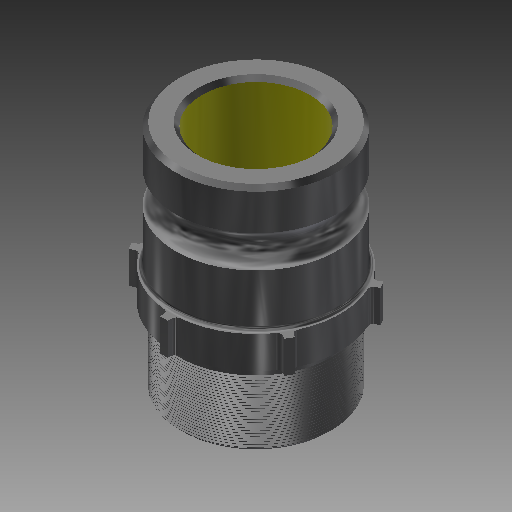
# Autodesk Inventor part: banjo male cam
Saved by Autodesk Inventor 2017 (Build 210142000, 142)
## iProperties
Created: 2013-09-06
Part Number: banjo male cam
Material: GFRP
Document SubType Name: Modeling
Designer: mrister
Density: 1.75 g/cm^3
Description: Cam Lock - 2" Male Adapter x Male Thr'd, (BANJO 200F)
Engineer: mrister
Mass: 751.241 g
Surface Area: 358.727 cm^2
Volume: 92.9754 cm^3
Appearance: Rubber - Black - Version 1.1
Author: mrister
Autodesk Inventor part; units mm, degrees
ref_plane "YZ Plane" through (0, 0, 0) normal (1, 0, 0) x (0, 1, 0)
ref_plane "XZ Plane" through (0, 0, 0) normal (0, 1, 0) x (-1, 0, 0)
ref_plane "XY Plane" through (0, 0, 0) normal (0, 0, 1) x (1, 0, 0)
sketch "Sketch1" plane through (0, 0, 0) normal (0, 0, 1) x (1, 0, 0)
  line L0 (-31.75, 0) -> (-31.75, 20.6375)
  arc A0 (-31.75, 20.6375) -> (-31.75, 33.3375) centre (-33.6021, 26.9875) ccw
  line L1 (-31.75, 33.3375) -> (-31.75, 49.2125)
  line L2 (-31.75, 49.2125) -> (-21.4313, 49.2125)
  line L3 (-21.4313, 49.2125) -> (-21.4312, 0)
  line L4 (-21.4312, 0) -> (-31.75, 0)
  line L5 (-21.4312, 0) -> (0, 0) construction
  line L6 (-31.75, 0) -> (-33.3375, 0)
  line L7 (-33.3375, 0) -> (-33.3375, -12.7)
  line L8 (-33.3375, -12.7) -> (-30.1625, -12.7)
  line L9 (-30.1625, -12.7) -> (-30.1625, -42.8625)
  line L10 (-30.1625, -42.8625) -> (-21.4312, -42.8625)
  line L11 (-21.4312, -42.8625) -> (-21.4312, 0)
  line L12 (0, -61.2775) -> (0, 67.6275) projected
  point P0 (-26.9875, 26.9875)
  dimension "d2" = 49.2125
  dimension "d5" = 12.7
  dimension "d28" = 21.4312
  dimension "d29" = 22.225
  dimension "d30" = 26.9875
  dimension "d31" = 31.75
  dimension "d32" = 30.1625
  dimension "d33" = 33.3375
  dimension "d34" = 92.075
  dimension "d35" = 30.1625
  constraints: 24 end point, 6 parallel, 3 collinear, 3 point on circle, 2 perpendicular, 1 centre point, 1 coincident, 1 horizontal, 1 vertical
  measures "d2" distance between parallel lines of L2 L4
  measures "d5" distance of L0.end L1.start
  measures "d28" distance from line of point (0, 0) L3
  measures "d29" distance from line of A0.centre L2
  measures "d30" horizontal distance of point (0, 0) point (-26.988, 26.987)
  measures "d31" distance from line of point (0, 0) L1
  measures "d32" distance from line of point (0, 0) L9
  measures "d33" distance from line of L5.end L7
  measures "d34" distance between parallel lines of L2 L10
  measures "d35" distance of L8.end L9.end
revolve "Revolution1" add sketch "Sketch1" angle 360 about axis through (0, -10, 0) along (0, 1, 0)
sketch "Sketch4" plane through (0, 0, 0) normal (0, 1, 0) x (-1, 0, 0)
  line L0 (-1.5875, 36.4747) -> (1.5875, 36.4747)
  line L1 (1.5875, 36.4747) -> (1.5875, 33.2997)
  line L2 (1.5875, 33.2997) -> (-1.5875, 33.2997)
  line L3 (-1.5875, 33.2997) -> (-1.5875, 36.4747)
  line L4 (0, 33.2997) -> (0, 0) construction
  circle A0 centre (0, 0) radius 33.3375 construction
  line L5 (-32.3818, 16.8625) -> (-30.7943, 19.6122)
  line L6 (-30.7943, 19.6122) -> (-28.0446, 18.0247)
  line L7 (-28.0446, 18.0247) -> (-29.6321, 15.275)
  line L8 (-29.6321, 15.275) -> (-32.3818, 16.8625)
  line L9 (-30.7943, -19.6122) -> (-32.3818, -16.8625)
  line L10 (-32.3818, -16.8625) -> (-29.6321, -15.275)
  line L11 (-29.6321, -15.275) -> (-28.0446, -18.0247)
  line L12 (-28.0446, -18.0247) -> (-30.7943, -19.6122)
  line L13 (1.5875, -36.4747) -> (-1.5875, -36.4747)
  line L14 (-1.5875, -36.4747) -> (-1.5875, -33.2997)
  line L15 (-1.5875, -33.2997) -> (1.5875, -33.2997)
  line L16 (1.5875, -33.2997) -> (1.5875, -36.4747)
  line L17 (32.3818, -16.8625) -> (30.7943, -19.6122)
  line L18 (30.7943, -19.6122) -> (28.0446, -18.0247)
  line L19 (28.0446, -18.0247) -> (29.6321, -15.275)
  line L20 (29.6321, -15.275) -> (32.3818, -16.8625)
  line L21 (30.7943, 19.6122) -> (32.3818, 16.8625)
  line L22 (32.3818, 16.8625) -> (29.6321, 15.275)
  line L23 (29.6321, 15.275) -> (28.0446, 18.0247)
  line L24 (28.0446, 18.0247) -> (30.7943, 19.6122)
  point P0 (-28.8384, 16.6498)
  point P1 (-28.8384, -16.6498)
  point P2 (0, -33.2997)
  point P3 (28.8384, -16.6498)
  point P4 (28.8384, 16.6498)
  dimension "d36" = 3.175
  dimension "d38" = 3.175
  dimension "d41" = 360
  constraints: 50 end point, 2 parallel, 1 horizontal, 1 midpoint, 1 perpendicular, 1 vertical, 57 other
  measures "d36" distance of L0.start L0.end
  measures "d38" distance of L0.end L1.end
extrude "Extrusion3" add sketch "Sketch4" against normal blind 12.7
chamfer "Chamfer3" distance 1.5875 angle 45 4 edges at (31.75, 49.2125, 0) (21.4313, 49.2125, 0) (30.1625, -42.8625, 0) (21.4312, -42.8625, 0)
fillet "Fillet2" radius 1.5875 14 edges at (30.1625, -12.7, 0) (31.75, 0, 0) (29.6321, -6.35, 15.275) (28.0446, -6.35, -18.0247) (1.5875, -6.35, -33.2997) (29.6321, -6.35, -15.275) (28.0446, -6.35, 18.0247) (1.5875, -6.35, 33.2997) (-1.5875, -6.35, 33.2997) (-28.0446, -6.35, 18.0247) (-29.6321, -6.35, -15.275) (-29.6321, -6.35, 15.275) (-28.0446, -6.35, -18.0247) (-1.5875, -6.35, -33.2997)
sketch "Sketch5" plane through (0, 0, 0) normal (0, 0, 1) x (1, 0, 0)
  line L0 (-30.1625, -41.275) -> (-30.1625, -14.2875) projected
  line L1 (-29.3687, -54.3166) -> (-30.1625, -54.7134)
  line L2 (-30.1625, -54.7134) -> (-30.1625, -53.9197)
  line L3 (-29.3687, -54.3166) -> (-30.1625, -54.3166) construction
  line L4 (-29.3687, -54.3166) -> (-30.1625, -53.9197)
  point P0 (0, 0)
  dimension "d49" = 0.7937
  dimension "d51" = 0.7937
  constraints: 8 end point, 2 collinear, 1 horizontal, 1 midpoint
  measures "d49" distance of L1.end L2.end
  measures "d51" distance of L1.start L3.end
coil "Coil1" sketch "Sketch5" operation cut axis through (0, -10, 0) along (0, 1, 0) pitch 0.9525 turns 40 hand right
equation "\"d51\" = d49"
body "Solid1"
